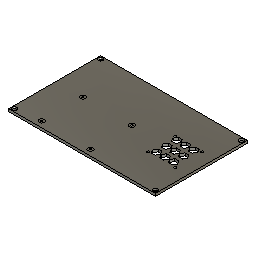
module_lid v2 (Autodesk Fusion 360 design; units mm, degrees)
Autodesk Fusion 360 part; units mm, degrees
sketch "Sketch1" plane through (0, 0, 0) normal (0, 0, 1) x (1, 0, 0)
  line L0 (0, 0) -> (174, 0)
  line L1 (174, 0) -> (174, 109)
  line L2 (174, 109) -> (0, 109)
  line L3 (0, 109) -> (0, 0)
  dimension "d1" = 174
  dimension "d2" = 109
  constraint horizontal L0
  constraint vertical L1
  constraint horizontal L2
  constraint vertical L3
  constraint coincident L0.start L3.end
  measures "d1" distance of L0.start L0.end
  measures "d2" distance of L0.start L2.end
extrude "Extrude1" add sketch "Sketch1" along normal blind 3 makes body 1
sketch "Sketch2" plane through (0, 0, 3) normal (0, 0, 1) x (-1, 0, 0)
  line L0 (0, -109) -> (0, 0)
  line L1 (0, 0) -> (-174, 0)
  line L2 (-174, 0) -> (-174, -109)
  line L3 (-174, -109) -> (0, -109)
  point P0 (-3.5, -3.5)
  point P1 (-3.5, -105.5)
  point P2 (-170.5, -105.5)
  point P3 (-170.5, -3.5)
hole "Hole1" at (170.5, 3.5, 3) at (3.5, 105.5, 3) at (3.5, 3.5, 3) at (170.5, 105.5, 3) direction (0, 0, -1) diameter 3.4 depth 6 tip angle 180 countersink diameter 5.75 countersink angle 90 bodies 1
sketch "Sketch6" plane through (0, 0, 3) normal (0, 0, 1) x (-1, 0, 0)
  circle A0 centre (-3.5, -3.5) radius 2.875
  circle A1 centre (-170.5, -3.5) radius 2.875
  circle A2 centre (-3.5, -105.5) radius 2.875
  circle A3 centre (-170.5, -105.5) radius 2.875
  line L0 (0, -109) -> (0, 0)
  line L1 (0, 0) -> (-174, 0)
  line L2 (-174, 0) -> (-174, -109)
  line L3 (-174, -109) -> (0, -109)
  circle A4 centre (-90, -7) radius 3
  circle A5 centre (-90, -56) radius 3
  circle A6 centre (-32, -7) radius 3
  circle A7 centre (-32, -56) radius 3
  point P0 (-32, -7)
  point P1 (-32, -56)
  point P2 (-90, -7)
  point P3 (-90, -56)
  dimension "d24" = 6
  dimension "d25" = 6
  dimension "d26" = 6
  dimension "d27" = 6
  constraint coincident P2 A4.centre
  constraint coincident P3 A5.centre
  constraint coincident P0 A6.centre
  constraint coincident P1 A7.centre
  measures "d24" diameter of A4
  measures "d25" diameter of A5
  measures "d26" diameter of A6
  measures "d27" diameter of A7
extrude "Extrude3" add sketch "Sketch6" against normal blind 7 separate body contours A4 | A5 | A6 | A7 makes body 2 at (87.0149, 7.2987, -1.6667) makes body 3 at (29.0149, 7.2987, -1.6667) makes body 4 at (89.0445, 53.1562, -1.6667) makes body 5 at (29.0149, 56.2987, -1.6667)
sketch "Sketch7" plane through (0, 0, -4) normal (0, 0, -1) x (1, 0, 0)
  circle A0 centre (90, -56) radius 3
  point P0 (90, -56)
  point P1 (90, -7)
  point P2 (32, -7)
  point P3 (32, -56)
  constraint coincident P0 A0.centre
  constraint vertical P0 P1
  constraint horizontal P1 P2
  constraint vertical P2 P3
hole "Hole2" at (90, 56, -4) at (90, 7, -4) at (32, 56, -4) at (32, 7, -4) direction (0, 0, 1) diameter 2.1 depth 14 tip angle 180 bodies 1 2 3 4 5
sketch "Sketch8" plane through (0, 0, 0) normal (0, 0, -1) x (1, 0, 0)
  circle A0 centre (32, -56) radius 1.05
  circle A1 centre (90, -56) radius 1.05
  circle A2 centre (90, -7) radius 1.05
  circle A3 centre (32, -7) radius 1.05
  circle A4 centre (3.5, -3.5) radius 1.7
  circle A5 centre (170.5, -3.5) radius 1.7
  circle A6 centre (3.5, -105.5) radius 1.7
  circle A7 centre (170.5, -105.5) radius 1.7
  line L0 (0, 0) -> (0, -109)
  line L1 (0, -109) -> (174, -109)
  line L2 (174, -109) -> (174, 0)
  line L3 (174, 0) -> (0, 0)
  line L4 (127, -38.5) -> (159, -38.5)
  line L5 (159, -38.5) -> (159, -70.5)
  line L6 (159, -70.5) -> (127, -70.5)
  line L7 (127, -70.5) -> (127, -38.5)
  line L8 (127, -38.5) -> (159, -70.5) construction
  line L9 (159, -38.5) -> (127, -70.5) construction
  point P0 (143, -54.5)
  point P1 (143, -54.5)
  dimension "d33" = 32
  dimension "d34" = 32
  constraint horizontal L4
  constraint perpendicular L4 L5
  constraint parallel L4 L6
  constraint parallel L5 L7
  constraint coincident L8 P1
  constraint coincident L9 P1
  constraint coincident P1 P0
  measures "d33" distance of L5.end L6.end
  measures "d34" distance of L4.end L5.end
hole "Hole3" at (159, 70.5, 0) at (127, 38.5, 0) at (127, 70.5, 0) at (159, 38.5, 0) direction (0, 0, 1) diameter 2.75 depth 14 tip angle 180 bodies 1
sketch "Sketch9" plane through (0, 0, 0) normal (0, 0, -1) x (1, 0, 0)
  circle A0 centre (127, -70.5) radius 1.375
  circle A1 centre (159, -70.5) radius 1.375
  circle A2 centre (127, -38.5) radius 1.375
  circle A3 centre (159, -38.5) radius 1.375
  circle A4 centre (32, -56) radius 1.05
  circle A5 centre (90, -56) radius 1.05
  circle A6 centre (90, -7) radius 1.05
  circle A7 centre (32, -7) radius 1.05
  circle A8 centre (3.5, -3.5) radius 1.7
  circle A9 centre (170.5, -3.5) radius 1.7
  circle A10 centre (3.5, -105.5) radius 1.7
  circle A11 centre (170.5, -105.5) radius 1.7
  line L0 (0, 0) -> (0, -109)
  line L1 (0, -109) -> (174, -109)
  line L2 (174, -109) -> (174, 0)
  line L3 (174, 0) -> (0, 0)
  line L4 (149.8625, -63.3271) -> (147.5531, -67.3271)
  line L5 (147.5531, -67.3271) -> (149.8625, -71.3271)
  line L6 (149.8625, -71.3271) -> (154.4814, -71.3271)
  line L7 (154.4814, -71.3271) -> (156.7908, -67.3271)
  line L8 (156.7908, -67.3271) -> (154.4814, -63.3271)
  line L9 (154.4814, -63.3271) -> (149.8625, -63.3271)
  line L10 (139.8625, -71.3271) -> (144.4814, -71.3271)
  line L11 (144.4814, -71.3271) -> (146.7908, -67.3271)
  line L12 (146.7908, -67.3271) -> (144.4814, -63.3271)
  line L13 (144.4814, -63.3271) -> (139.8625, -63.3271)
  line L14 (139.8625, -63.3271) -> (137.5531, -67.3271)
  line L15 (137.5531, -67.3271) -> (139.8625, -71.3271)
  line L16 (129.8625, -71.3271) -> (134.4814, -71.3271)
  line L17 (134.4814, -71.3271) -> (136.7908, -67.3271)
  line L18 (136.7908, -67.3271) -> (134.4814, -63.3271)
  line L19 (134.4814, -63.3271) -> (129.8625, -63.3271)
  line L20 (129.8625, -63.3271) -> (127.5531, -67.3271)
  line L21 (127.5531, -67.3271) -> (129.8625, -71.3271)
  line L22 (149.8625, -59.3271) -> (154.4814, -59.3271)
  line L23 (154.4814, -59.3271) -> (156.7908, -55.3271)
  line L24 (156.7908, -55.3271) -> (154.4814, -51.3271)
  line L25 (154.4814, -51.3271) -> (149.8625, -51.3271)
  line L26 (149.8625, -51.3271) -> (147.5531, -55.3271)
  line L27 (147.5531, -55.3271) -> (149.8625, -59.3271)
  line L28 (139.8625, -59.3271) -> (144.4814, -59.3271)
  line L29 (144.4814, -59.3271) -> (146.7908, -55.3271)
  line L30 (146.7908, -55.3271) -> (144.4814, -51.3271)
  line L31 (144.4814, -51.3271) -> (139.8625, -51.3271)
  line L32 (139.8625, -51.3271) -> (137.5531, -55.3271)
  line L33 (137.5531, -55.3271) -> (139.8625, -59.3271)
  line L34 (129.8625, -59.3271) -> (134.4814, -59.3271)
  line L35 (134.4814, -59.3271) -> (136.7908, -55.3271)
  line L36 (136.7908, -55.3271) -> (134.4814, -51.3271)
  line L37 (134.4814, -51.3271) -> (129.8625, -51.3271)
  line L38 (129.8625, -51.3271) -> (127.5531, -55.3271)
  line L39 (127.5531, -55.3271) -> (129.8625, -59.3271)
  line L40 (149.8625, -47.3271) -> (154.4814, -47.3271)
  line L41 (154.4814, -47.3271) -> (156.7908, -43.3271)
  line L42 (156.7908, -43.3271) -> (154.4814, -39.3271)
  line L43 (154.4814, -39.3271) -> (149.8625, -39.3271)
  line L44 (149.8625, -39.3271) -> (147.5531, -43.3271)
  line L45 (147.5531, -43.3271) -> (149.8625, -47.3271)
  line L46 (139.8625, -47.3271) -> (144.4814, -47.3271)
  line L47 (144.4814, -47.3271) -> (146.7908, -43.3271)
  line L48 (146.7908, -43.3271) -> (144.4814, -39.3271)
  line L49 (144.4814, -39.3271) -> (139.8625, -39.3271)
  line L50 (139.8625, -39.3271) -> (137.5531, -43.3271)
  line L51 (137.5531, -43.3271) -> (139.8625, -47.3271)
  line L52 (129.8625, -47.3271) -> (134.4814, -47.3271)
  line L53 (134.4814, -47.3271) -> (136.7908, -43.3271)
  line L54 (136.7908, -43.3271) -> (134.4814, -39.3271)
  line L55 (134.4814, -39.3271) -> (129.8625, -39.3271)
  line L56 (129.8625, -39.3271) -> (127.5531, -43.3271)
  line L57 (127.5531, -43.3271) -> (129.8625, -47.3271)
  point P0 (152.172, -67.3271)
  point P1 (142.238, -62.3661)
  point P2 (132.9985, -66.7092)
  dimension "d39" = 4
  dimension "d44" = -10
  dimension "d45" = 12
  measures "d39" distance of P0 L9
extrude "Extrude4" cut sketch "Sketch9" against normal blind 1000 contours L4 L5 L6 L7 L8 L9 | L10 L11 L12 L13 L14 L15 | L16 L17 L18 L19 L20 L21 | L22 L23 L24 L25 L26 L27 | L28 L29 L30 L31 L32 L33 | L34 L35 L36 L37 L38 L39 | L40 L41 L42 L43 L44 L45 | L46 L47 L48 L49 L50 L51 | L52 L53 L54 L55 L56 L57 bodies 1
